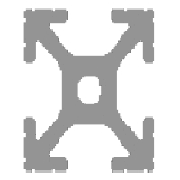
# Autodesk Inventor part: 1010_80_20
Saved by Autodesk Inventor 2012 (Build 160160000, 160)
## iProperties
Created: 2012-10-25
Part Number: 1010_80_20
Material: Aluminum-6061
Description: 1x1 T-Slot
Document SubType Name: Modeling
Standard: ANSI
Designer: Andrew G. Meyer
Standards Organization: ANSI
Language: en-US
Size Designation: 1010_80_20
Categories: <MemberInstance><Categories><Category DisplayName="Structural Shapes" InternalName="089c4875-fa83-4c05-b084-43b9cc11f5ed" Mnemonic="GRDR"><CategoryParameter DisplayName="Custom Base Point" InternalName="4f1d1b73-316d-484b-a3df-9cbabb16eb77" Mnemonic="shpBasePoint"/><CategoryParameter DisplayName="FG Authored" InternalName="9c666724-f362-4ea7-ac62-f6a007de5c69" Mnemonic="shpFGAuto"/><CategoryParameter DisplayName="Legacy Member ID" InternalName="340afe4f-75d7-48d3-ab7d-943f3c3da468" Mnemonic="LegacyMemberID"/><CategoryParameter DisplayName="Base Length" InternalName="42e34263-8f20-4d0e-ad48-bf1385b87c24" Mnemonic="shplen"/><CategoryParameter DisplayName="Distance of the Center of Gravity X-X" InternalName="26c9bdb8-9c79-4b4f-a92e-8e197583c9c4" Mnemonic="grcendistX"/><CategoryParameter DisplayName="Distance of the Center of Gravity Y-Y" InternalName="bcc4fb17-7af4-436a-8f8c-d0aa3b0248c5" Mnemonic="grcendistY"/><CategoryParameter DisplayName="Torsional Rigidity Modulus" InternalName="26c1ec35-5026-4c63-ad0a-751cf684a536" Mnemonic="torrigmod"/><CategoryParameter DisplayName="Torsional Section Modulus" InternalName="7c55a8dc-8844-49f9-a867-cc677b30ec9a" Mnemonic="torsecmod"/><CategoryParameter DisplayName="Coefficient of Shear Displacement" InternalName="de4c90c6-aaa8-468f-a335-6737b311b5d3" Mnemonic="shdispc"/><CategoryParameter DisplayName="Section Area" InternalName="1ff91680-64b0-4202-b9a3-7fd3f94bba3b" Mnemonic="secarea"/><CategoryParameter DisplayName="Moment of Inertia (x)" InternalName="4cd780bc-73d7-43ac-917a-579e5cbd684d" Mnemonic="inermomx"/><CategoryParameter DisplayName="Moment of Inertia (y)" InternalName="4b9f58ea-bced-460e-81ea-3d29ca5a49e3" Mnemonic="inermomy"/><CategoryParameter DisplayName="Section Module (x)" InternalName="72cfad18-cf51-4ed4-aaa7-c6b224f8419f" Mnemonic="secmodx"/><CategoryParameter DisplayName="Section Module (y)" InternalName="59eaa5e9-d227-48dc-b6c1-6920f96e0f95" Mnemonic="secmody"/><CategoryParameter DisplayName="Radius of Gyration (x)" InternalName="25778675-03e9-40c1-b6a8-4a9ed693320d" Mnemonic="gyrradx"/><CategoryParameter DisplayName="Radius of Gyration (y)" InternalName="bfa18ebe-1636-4dbe-8d42-b263e0b73184" Mnemonic="gyrrady"/><CategoryParameter DisplayName="Shape Thickness" InternalName="d109cf76-8eb4-42fc-9800-4409734adc67" Mnemonic="shpthick"/><CategoryParameter DisplayName="Second Shape Thickness" InternalName="9251a8e1-85fd-4e47-af99-afdb762317d9" Mnemonic="shpthick2"/><CategoryParameter DisplayName="Shape Width" InternalName="7c717d54-a18f-4666-b4d4-573cce22c62c" Mnemonic="shpwdth"/><CategoryParameter DisplayName="Shape Height" InternalName="50274e7d-5ac0-4796-92cb-c59e54983c67" Mnemonic="shpheig"/><CategoryParameter DisplayName="Mass per Length Unit" InternalName="0bb95a10-148f-4027-a459-38d7b056702a" Mnemonic="shpmass"/><CategoryParameter DisplayName="Section Designation" InternalName="5a64d034-428d-49c8-ba32-7619764de20f" Mnemonic="shpdes"/><Category DisplayName="Square/Rectangular Tubes" InternalName="afc8e2d8-05d6-4609-8807-f98a9b7d2ed0" Mnemonic="SQRSHP"><CategoryParameter DisplayName="Moment of Inertia (x)" InternalName="8c4637b6-6b69-4878-9d5d-26a32185d655" Mnemonic="inermomx"/><CategoryParameter DisplayName="Moment of Inertia (y)" InternalName="55ec8510-8276-4c45-8f10-594e0fee7eb3" Mnemonic="inermomy"/><CategoryParameter DisplayName="Section Module (x)" InternalName="50d965a6-04bf-46b9-8ace-861858d348e6" Mnemonic="secmodx"/><CategoryParameter DisplayName="Section Module (y)" InternalName="5106aeac-54a2-4159-a9af-8933dd39dba2" Mnemonic="secmody"/><CategoryParameter DisplayName="Section Area" InternalName="2f7f79dd-983c-4263-802a-5b6a1495fdc5" Mnemonic="secarea"/><CategoryParameter DisplayName="Radius of Gyration (x)" InternalName="56c89926-a299-4389-a862-ac94c9691272" Mnemonic="gyrradx"/><CategoryParameter DisplayName="Radius of Gyration (y)" InternalName="fa48a7f5-f030-40f9-a60b-de8a845b7104" Mnemonic="gyrrady"/><CategoryParameter DisplayName="Shape Width" InternalName="8c8a1782-5e80-4d77-858b-304b1c0ad1fd" Mnemonic="shpwdth"/><CategoryParameter DisplayName="Shape Thickness" InternalName="52712fc5-f4ee-4eda-b3f2-6fce82c26419" Mnemonic="shpthick"/><CategoryParameter DisplayName="Radius" InternalName="5d8d062c-e28e-41c1-98da-8e5fee36da1a" Mnemonic="shprad"/></Category></Category><Category DisplayName="DataType" InternalName="23b78d0f-2648-40c6-8793-ca6db495c9e8" Mnemonic="DATATYPE"><CategoryParameter DisplayName="DisplayName" InternalName="05415f3d-3907-474b-a020-eb9d644f4cf3" Mnemonic="DISPLAYNAME"/><CategoryParameter DisplayName="InternalName" InternalName="cf1d0246-76d9-4b4a-8305-fa0409afb5c1" Mnemonic="INTERNALNAME"/><CategoryParameter DisplayName="Folder Name" InternalName="3f06958e-8713-4116-9be7-ed6184ecc97b" Mnemonic="FOLDERNAME"/><CategoryParameter DisplayName="Family Version" InternalName="914462f6-6e19-4b14-ba84-155b9680b1d0" Mnemonic="FAMILYREVISION"/><CategoryParameter DisplayName="ClipFormat" InternalName="bc51e27b-3422-4e78-93ef-cec197ddf230" Mnemonic="CLIPFORMAT"/><CategoryParameter DisplayName="IsMetric" InternalName="e2385c5b-1ea4-4823-96a8-8de651266ec3" Mnemonic="ISMETRIC"/><CategoryParameter DisplayName="Description" InternalName="13903e3d-64b1-4950-80da-f627842ea37f" Mnemonic="DESCRIPTION"/><CategoryParameter DisplayName="StdsOrg" InternalName="8f5914e1-4693-403f-8ab5-d37768198c9d" Mnemonic="STDSORG"/><CategoryParameter DisplayName="Standard" InternalName="0c0a119c-1e12-4c84-803f-101930972f5e" Mnemonic="STANDARD"/><CategoryParameter DisplayName="Manufacturer" InternalName="cd6c7a72-a28a-4e50-99a9-2c7f4e13e5ad" Mnemonic="MANUFACTURER"/><CategoryParameter DisplayName="Member Revision" InternalName="a65d44b9-392f-4f4f-857b-e4b3d54996fe" Mnemonic="MEMBERREVISION"/><CategoryParameter DisplayName="Standard Revision" InternalName="91d5a463-65c2-4fde-b823-3b7fea5e8e17" Mnemonic="STANDARDREVISION"/><CategoryParameter DisplayName="Revision Guid" InternalName="45a75005-10b1-4dfc-8d6d-dfe629f0b93c" Mnemonic="REVISIONGUID"/><CategoryParameter DisplayName="Designation" InternalName="2675968c-4ce5-49e0-a4f5-552d29089031" Mnemonic="DESIGNATION"/><CategoryParameter DisplayName="FileName" InternalName="8b46a4cc-9585-4fed-90c3-899f57e09a73" Mnemonic="FILENAME"/><CategoryParameter DisplayName="Default Row" InternalName="2af9ec52-faaa-4026-b378-f9fa4afca842" Mnemonic="DEFAULTROW"/><Category DisplayName="Part" InternalName="c0e0b642-3bcb-4cc8-9e80-f96d35c4afa4" Mnemonic="PART"><CategoryParameter DisplayName="Material" InternalName="818a152a-d3c3-49ca-80ee-df7d91421b8e" Mnemonic="MATERIAL"/><CategoryParameter DisplayName="Material Key" InternalName="5c9a8adb-dd2b-4535-b97f-0a94a95fe41f" Mnemonic="MATERIALKEY"/><CategoryParameter DisplayName="Part Number" InternalName="016b6077-bfbe-49bd-92c9-d8d59c39c941" Mnemonic="PARTNUMBER"/><CategoryParameter DisplayName="Stock Number" InternalName="4dba7c1c-e26c-444e-836c-b08b433409a8" Mnemonic="STOCKNUMBER"/></Category></Category></Categories><FamilyTemplate Id="1010_80_20"><FamilyTemplateParameters><FamilyTemplateParameter ObjectType="kModelParameterObject" ValueType="xs:double" Id="12" ObjectReferenceKey="Length"/><FamilyTemplateParameter ObjectType="kPartComponentDefinitionObject" ValueType="xs:string" Id="23" SubObjectId="Material"/><FamilyTemplateParameter ObjectType="kPropertyObject" ValueType="xs:string" Id="26" ObjectReferenceKey="{32853F0F-3444-11d1-9E93-0060B03C1CA6}" SubObjectId="5"/><FamilyTemplateParameter ObjectType="kPropertyObject" ValueType="xs:string" Id="27" ObjectReferenceKey="{32853F0F-3444-11d1-9E93-0060B03C1CA6}" SubObjectId="52"/></FamilyTemplateParameters></FamilyTemplate><CategoryParameterMap><ParamToTemplateMap><ParamToTemplate CategoryParameter="//CategoryParameter[@InternalName='cf1d0246-76d9-4b4a-8305-fa0409afb5c1']" ConstantValue="d420446d-5aa0-4a6f-95a1-e316646d4d7a"/><ParamToTemplate CategoryParameter="//CategoryParameter[@InternalName='45a75005-10b1-4dfc-8d6d-dfe629f0b93c']" ConstantValue="273de972-af0a-4669-b29d-06cc7d807bd5"/><ParamToTemplate CategoryParameter="//CategoryParameter[@InternalName='3f06958e-8713-4116-9be7-ed6184ecc97b']" ConstantValue="1010_80_20"/><ParamToTemplate CategoryParameter="//CategoryParameter[@InternalName='8f5914e1-4693-403f-8ab5-d37768198c9d']" ConstantValue="ANSI"/><ParamToTemplate CategoryParameter="//CategoryParameter[@InternalName='0c0a119c-1e12-4c84-803f-101930972f5e']" ConstantValue="AISC"/><ParamToTemplate CategoryParameter="//CategoryParameter[@InternalName='91d5a463-65c2-4fde-b823-3b7fea5e8e17']" TemplateParameter="19"/><ParamToTemplate CategoryParameter="//CategoryParameter[@InternalName='cd6c7a72-a28a-4e50-99a9-2c7f4e13e5ad']" TemplateParameter="20"/><ParamToTemplate CategoryParameter="//CategoryParameter[@InternalName='13903e3d-64b1-4950-80da-f627842ea37f']" ConstantValue="1x1 T-Slot"/><ParamToTemplate CategoryParameter="//CategoryParameter[@InternalName='05415f3d-3907-474b-a020-eb9d644f4cf3']" ConstantValue="1010_80_20"/><ParamToTemplate CategoryParameter="//CategoryParameter[@InternalName='914462f6-6e19-4b14-ba84-155b9680b1d0']" ConstantValue="11"/><ParamToTemplate CategoryParameter="//CategoryParameter[@InternalName='bc51e27b-3422-4e78-93ef-cec197ddf230']" ConstantValue="CF_INVENTOR.STDPARTS"/><ParamToTemplate CategoryParameter="//CategoryParameter[@InternalName='e2385c5b-1ea4-4823-96a8-8de651266ec3']" ConstantValue="false"/><ParamToTemplate CategoryParameter="//CategoryParameter[@InternalName='2af9ec52-faaa-4026-b378-f9fa4afca842']" ConstantValue="1"/><ParamToTemplate CategoryParameter="//CategoryParameter[@InternalName='9c666724-f362-4ea7-ac62-f6a007de5c69']" ConstantValue="1"/><ParamToTemplate CategoryParameter="//CategoryParameter[@InternalName='8b46a4cc-9585-4fed-90c3-899f57e09a73']" ConstantValue="1-1010_80_20"/><ParamToTemplate CategoryParameter="//CategoryParameter[@InternalName='a65d44b9-392f-4f4f-857b-e4b3d54996fe']" ConstantValue="fcaa9394-dcdd-4557-997d-f25d4b9153c8"/><ParamToTemplate CategoryParameter="//CategoryParameter[@InternalName='a65d44b9-392f-4f4f-857b-e4b3d54996fe']" ConstantValue="fcaa9394-dcdd-4557-997d-f25d4b9153c8"/><ParamToTemplate CategoryParameter="//CategoryParameter[@InternalName='2675968c-4ce5-49e0-a4f5-552d29089031']" TemplateParameter="27"/><ParamToTemplate CategoryParameter="//CategoryParameter[@InternalName='42e34263-8f20-4d0e-ad48-bf1385b87c24']" TemplateParameter="12"/><ParamToTemplate CategoryParameter="//CategoryParameter[@InternalName='818a152a-d3c3-49ca-80ee-df7d91421b8e']" TemplateParameter="23"/><ParamToTemplate CategoryParameter="//CategoryParameter[@InternalName='016b6077-bfbe-49bd-92c9-d8d59c39c941']" TemplateParameter="26"/></ParamToTemplateMap></CategoryParameterMap></MemberInstance>
Mass: 19.709 g
Surface Area: 59.6867 cm^2
Volume: 7.2727 cm^3
Density: 2.71 g/cm^3
IsCustomPart: 1
Author: Andrew G. Meyer
Width: 1.000 in
Height: 1.000 in
Length: 11.000 in
G_L: 11.000 in
G_W: 1.000 in
G_H: 1.000 in
_CCFamilyDisplayName: 1010_80_20 - 1x1 T-Slot
_FrameMemberDoc: Frame Member File
_Version: 15.0.0
_GetPNFromCC: 1
Autodesk Inventor part; units mm, degrees
ref_plane "Start Plane" through (0, 0, -12.7) normal (0, 0, 1) x (1, 0, 0)
ref_plane "End Plane" through (0, 0, 266.7) normal (0, 0, 1) x (1, 0, 0)
sketch "Sketch" plane through (0, 0, 0) normal (0, 0, 1) x (1, 0, 0)
  arc A0 (-11.6332, 12.7) -> (-12.7, 11.6332) centre (-11.6332, 11.6332) ccw
  arc A1 (-5.3594, 10.5664) -> (-5.3594, 12.7) centre (-5.3594, 11.6332) ccw
  arc A2 (-12.7, 5.3594) -> (-10.5664, 5.3594) centre (-11.6332, 5.3594) ccw
  line L0 (-10.5664, 7.493) -> (-10.5664, 5.3594)
  line L1 (-7.493, 10.5664) -> (-5.3594, 10.5664)
  arc A3 (-9.6992, 7.8522) -> (-10.5664, 7.493) centre (-10.0584, 7.493) ccw
  arc A4 (-7.493, 10.5664) -> (-7.8522, 9.6992) centre (-7.493, 10.0584) ccw
  line L2 (-11.6332, 11.6332) -> (0, 0) construction
  line L3 (-5.8003, 3.9533) -> (-9.6992, 7.8522)
  line L4 (-7.8522, 9.6992) -> (-3.9533, 5.8003)
  arc A5 (-3.9533, 5.8003) -> (-2.6924, 5.278) centre (-2.6924, 7.0612) ccw
  arc A6 (-5.278, 2.6924) -> (-5.8003, 3.9533) centre (-7.0612, 2.6924) ccw
  arc A7 (0, 2.54) -> (-2.54, 0) centre (0, 0) ccw construction
  line L5 (0, 0) -> (-12.7, 0) construction
  line L6 (0, 12.7) -> (0, 0) construction
  arc A8 (-11.6332, 12.7) -> (-10.6172, 12.7) centre (-11.1252, 12.7) ccw
  arc A9 (-7.5692, 12.7) -> (-6.5532, 12.7) centre (-7.0612, 12.7) ccw
  arc A10 (-12.7, 10.6172) -> (-12.7, 11.6332) centre (-12.7, 11.1252) ccw
  arc A11 (-12.7, 6.5532) -> (-12.7, 7.5692) centre (-12.7, 7.0612) ccw
  line L7 (-12.7, 10.6172) -> (-12.7, 7.5692)
  line L8 (-12.7, 6.5532) -> (-12.7, 5.3594)
  line L9 (-10.6172, 12.7) -> (-7.5692, 12.7)
  line L10 (-6.5532, 12.7) -> (-5.3594, 12.7)
  circle A12 centre (0, 0) radius 2.54
  arc A13 (-12.7, -11.6332) -> (-11.6332, -12.7) centre (-11.6332, -11.6332) ccw
  line L11 (-12.7, -10.6172) -> (-12.7, -7.5692)
  arc A14 (-10.5664, -7.493) -> (-9.6992, -7.8522) centre (-10.0584, -7.493) ccw
  line L12 (-9.6992, -7.8522) -> (-5.8003, -3.9533)
  line L13 (-11.6332, -11.6332) -> (0, 0) construction
  line L14 (-3.9533, -5.8003) -> (-7.8522, -9.6992)
  arc A15 (-7.8522, -9.6992) -> (-7.493, -10.5664) centre (-7.493, -10.0584) ccw
  line L15 (-10.6172, -12.7) -> (-7.5692, -12.7)
  line L16 (-7.493, -10.5664) -> (-5.3594, -10.5664)
  arc A16 (-6.5532, -12.7) -> (-7.5692, -12.7) centre (-7.0612, -12.7) ccw
  line L17 (-6.5532, -12.7) -> (-5.3594, -12.7)
  arc A17 (-5.3594, -12.7) -> (-5.3594, -10.5664) centre (-5.3594, -11.6332) ccw
  arc A18 (-10.6172, -12.7) -> (-11.6332, -12.7) centre (-11.1252, -12.7) ccw
  arc A19 (-12.7, -11.6332) -> (-12.7, -10.6172) centre (-12.7, -11.1252) ccw
  arc A20 (-2.6924, -5.278) -> (-3.9533, -5.8003) centre (-2.6924, -7.0612) ccw
  arc A21 (-5.8003, -3.9533) -> (-5.278, -2.6924) centre (-7.0612, -2.6924) ccw
  line L18 (-10.5664, -7.493) -> (-10.5664, -5.3594)
  line L19 (-12.7, -6.5532) -> (-12.7, -5.3594)
  arc A22 (-10.5664, -5.3594) -> (-12.7, -5.3594) centre (-11.6332, -5.3594) ccw
  arc A23 (-12.7, -7.5692) -> (-12.7, -6.5532) centre (-12.7, -7.0612) ccw
  arc A24 (11.6332, -12.7) -> (12.7, -11.6332) centre (11.6332, -11.6332) ccw
  line L20 (10.6172, -12.7) -> (7.5692, -12.7)
  arc A25 (7.493, -10.5664) -> (7.8522, -9.6992) centre (7.493, -10.0584) ccw
  line L21 (7.8522, -9.6992) -> (3.9533, -5.8003)
  line L22 (11.6332, -11.6332) -> (0, 0) construction
  line L23 (5.8003, -3.9533) -> (9.6992, -7.8522)
  arc A26 (9.6992, -7.8522) -> (10.5664, -7.493) centre (10.0584, -7.493) ccw
  line L24 (12.7, -10.6172) -> (12.7, -7.5692)
  line L25 (10.5664, -7.493) -> (10.5664, -5.3594)
  arc A27 (12.7, -6.5532) -> (12.7, -7.5692) centre (12.7, -7.0612) ccw
  line L26 (12.7, -6.5532) -> (12.7, -5.3594)
  arc A28 (12.7, -5.3594) -> (10.5664, -5.3594) centre (11.6332, -5.3594) ccw
  arc A29 (12.7, -10.6172) -> (12.7, -11.6332) centre (12.7, -11.1252) ccw
  arc A30 (11.6332, -12.7) -> (10.6172, -12.7) centre (11.1252, -12.7) ccw
  arc A31 (5.278, -2.6924) -> (5.8003, -3.9533) centre (7.0612, -2.6924) ccw
  arc A32 (3.9533, -5.8003) -> (2.6924, -5.278) centre (2.6924, -7.0612) ccw
  line L27 (7.493, -10.5664) -> (5.3594, -10.5664)
  line L28 (6.5532, -12.7) -> (5.3594, -12.7)
  arc A33 (5.3594, -10.5664) -> (5.3594, -12.7) centre (5.3594, -11.6332) ccw
  arc A34 (7.5692, -12.7) -> (6.5532, -12.7) centre (7.0612, -12.7) ccw
  arc A35 (12.7, 11.6332) -> (11.6332, 12.7) centre (11.6332, 11.6332) ccw
  line L29 (12.7, 10.6172) -> (12.7, 7.5692)
  arc A36 (10.5664, 7.493) -> (9.6992, 7.8522) centre (10.0584, 7.493) ccw
  line L30 (9.6992, 7.8522) -> (5.8003, 3.9533)
  line L31 (11.6332, 11.6332) -> (0, 0) construction
  line L32 (3.9533, 5.8003) -> (7.8522, 9.6992)
  arc A37 (7.8522, 9.6992) -> (7.493, 10.5664) centre (7.493, 10.0584) ccw
  line L33 (10.6172, 12.7) -> (7.5692, 12.7)
  line L34 (7.493, 10.5664) -> (5.3594, 10.5664)
  arc A38 (6.5532, 12.7) -> (7.5692, 12.7) centre (7.0612, 12.7) ccw
  line L35 (6.5532, 12.7) -> (5.3594, 12.7)
  arc A39 (5.3594, 12.7) -> (5.3594, 10.5664) centre (5.3594, 11.6332) ccw
  arc A40 (10.6172, 12.7) -> (11.6332, 12.7) centre (11.1252, 12.7) ccw
  arc A41 (12.7, 11.6332) -> (12.7, 10.6172) centre (12.7, 11.1252) ccw
  arc A42 (2.6924, 5.278) -> (3.9533, 5.8003) centre (2.6924, 7.0612) ccw
  arc A43 (5.8003, 3.9533) -> (5.278, 2.6924) centre (7.0612, 2.6924) ccw
  line L36 (10.5664, 7.493) -> (10.5664, 5.3594)
  line L37 (12.7, 6.5532) -> (12.7, 5.3594)
  arc A44 (10.5664, 5.3594) -> (12.7, 5.3594) centre (11.6332, 5.3594) ccw
  arc A45 (12.7, 7.5692) -> (12.7, 6.5532) centre (12.7, 7.0612) ccw
  line L38 (-2.6924, 5.278) -> (2.6924, 5.278)
  line L39 (-5.278, 2.6924) -> (-5.278, -2.6924)
  line L40 (-2.6924, -5.278) -> (2.6924, -5.278)
  line L41 (5.278, -2.6924) -> (5.278, 2.6924)
  point P0 (0, 0)
  point P1 (0, 0)
  dimension "d2" = 2.1336
  dimension "d3" = 6.2738
  dimension "d4" = 6.2738
  dimension "d5" = 1.0668
  dimension "d6" = 2.1336
  dimension "d7" = 2.1336
  dimension "d8" = 1.016
  dimension "d9" = 1.016
  dimension "d10" = 135
  dimension "d11" = 2.667
  dimension "d12" = 4.572
  dimension "d13" = 4.572
  dimension "d14" = 2.667
  dimension "d15" = 5.08
  dimension "d16" = 45
  dimension "d19" = 45
  dimension "d20" = 0.508
  dimension "d21" = 4.572
  dimension "d22" = 1.016
  dimension "d23" = 4.572
  dimension "d24" = 1.016
  dimension "d25" = 0.508
  dimension "d26" = 0.508
  dimension "d27" = 0.508
  dimension "d28" = 12.7
  dimension "d37" = 360
  dimension "d47" = 10.5664
  dimension "d48" = 12.7
  constraints: 90 point on circle, 88 end point, 46 centre point, 26 tangent, 18 point on line, 5 coincident, 4 perpendicular, 2 equal radius, 2 parallel, 1 horizontal, 1 horizontal alignment, 1 vertical alignment, 214 other
  measures "d2" diameter of A0
  measures "d3" distance of A0.centre A2.centre
  measures "d4" distance of A1.centre A0.centre
  measures "d5" radius of A1
  measures "d6" horizontal distance of A1.centre A4.centre
  measures "d7" vertical distance of A3.centre A2.centre
  measures "d8" diameter of A3
  measures "d9" diameter of A4
  measures "d10" angle of L1 L2
  measures "d11" vertical distance of A2.centre A6.centre
  measures "d12" horizontal distance of A2.centre A6.centre
  measures "d13" vertical distance of A1.centre A5.centre
  measures "d14" horizontal distance of A1.centre A5.centre
  measures "d15" diameter of A7
  measures "d16" angle of L2 L6
  measures "d19" angle of L2 L5
  measures "d20" horizontal distance of A8.centre A0.centre
  measures "d21" horizontal distance of A9.centre A0.centre
  measures "d22" diameter of A9
  measures "d23" vertical distance of A0.centre A11.centre
  measures "d24" diameter of A11
  measures "d25" vertical distance of A0.centre A10.centre
  measures "d26" radius of A10
  measures "d27" radius of A8
  measures "d28" vertical distance of L2.end L10.end
  measures "d47" distance from line of A12.centre L27
  measures "d48" distance from line of A12.centre L37
extrude "Body" add sketch "Sketch" along normal up to surface (279.4 mm away) from surface at -12.7
sketch "Sketch2" plane through (0, 0, 0) normal (0, 0, 1) x (1, 0, 0)
  line L0 (0, 0) -> (10, 0)
ref_plane "Work Plane3" through (0, 0, 0) normal (0, -1, 0) x (1, 0, 0)
sketch "Sketch3" plane through (0, 0, 0) normal (0, -1, 0) x (1, 0, 0)
  line L0 (-2, -12.7) -> (12, -12.7)
  line L1 (-2, 266.7) -> (12, 266.7)
  dimension "d60" = 279.4
  measures "d60" distance between parallel lines of L0 L1
ref_plane "Work Plane4" through (10.6172, 0, 266.7) normal (0, 0, 1) x (1, 0, 0)
split "Split1" plane through (10.6172, 0, 266.7) removes the side toward (0, 0, 1)
ref_plane "Work Plane5" through (1193.8, -10.6172, -12.7) normal (0, 0, -1) x (-1, 0, 0)
split "Split2" plane through (1193.8, -10.6172, -12.7) removes the side toward (0, 0, -1)
ref_plane "Work Plane6" through (7.5692, -279.4, -12.7) normal (0, 0, -1) x (-1, 0, 0)
split "Split3" plane through (7.5692, -279.4, -12.7) removes the side toward (0, 0, -1)
equation "\"d3\" = d4"
equation "\"d6\" = d7"
equation "\"d11\" = d14"
equation "\"d12\" = d13"
equation "\"d23\" = d21"
equation "\"d24\" = d30"
equation "\"d26\" = 0.5 * d24"
equation "\"d27\" = 0.5 * d22"
equation "\"Width\" = 2 * d28"
equation "\"Height\" = 2 * d48"
equation "\"G_OFFSET_START\" = 12.7"
equation "\"G_OFFSET_END\" = -12.7"
equation "\"d55\" = -G_OFFSET_START"
equation "\"d56\" = Length + G_OFFSET_END"
equation "\"G_L\" = 279.4"
equation "\"d30\" = 1.016"
equation "\"Length\" = 279.4"
body "Solid1"
